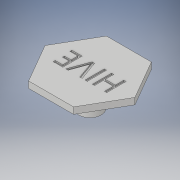
# Autodesk Inventor part: stand
Saved by Autodesk Inventor 2019 (Build 230136000, 136)
## iProperties
Created: 2018-06-01
Part Number: stand
Material: Generic
Document SubType Name: Modeling
Designer: HIVE
Density: 1 g/cm^3
Appearance: Default
Author: HIVE
## iProperties of the stored document stand_3DPrint.ipt
Created: 2018-06-01
Part Number: stand_3DPrint
Material: Generic
Document SubType Name: Modeling
Designer: HIVE
Density: 1 g/cm^3
Appearance: Default
Author: HIVE
Autodesk Inventor part; units mm, degrees
ref_plane "YZ Plane" through (0, 0, 0) normal (1, 0, 0) x (0, 1, 0)
ref_plane "XZ Plane" through (0, 0, 0) normal (0, 1, 0) x (-1, 0, 0)
ref_plane "XY Plane" through (0, 0, 0) normal (0, 0, 1) x (1, 0, 0)
sketch "Sketch1" plane through (0, 0, 0) normal (0, 1, 0) x (-1, 0, 0)
  circle A0 centre (0, 0) radius 35
  line L0 (17.5, -30.3109) -> (-17.5, -30.3109)
  line L1 (-17.5, -30.3109) -> (-35, 0)
  line L2 (-35, 0) -> (-17.5, 30.3109)
  line L3 (-17.5, 30.3109) -> (17.5, 30.3109)
  line L4 (17.5, 30.3109) -> (35, 0)
  line L5 (35, 0) -> (17.5, -30.3109)
  line L6 (16.3453, -28.3109) -> (-16.3453, -28.3109)
  line L7 (-16.3453, -28.3109) -> (-32.6906, 0)
  line L8 (-32.6906, 0) -> (-16.3453, 28.3109)
  line L9 (-16.3453, 28.3109) -> (16.3453, 28.3109)
  line L10 (16.3453, 28.3109) -> (32.6906, 0)
  line L11 (32.6906, 0) -> (16.3453, -28.3109)
  line L12 (0, 0) -> (-17.5, -30.3109)
  circle A1 centre (0, 0) radius 8.75
  line L13 (-22.7839, 7.707) -> (22.7839, 7.707) construction
  line L14 (22.7839, 7.707) -> (22.7839, -7.707) construction
  line L15 (22.7839, -7.707) -> (-22.7839, -7.707) construction
  line L16 (-22.7839, -7.707) -> (-22.7839, 7.707) construction
  line L17 (0, 0) -> (0, -28.3109) construction
  line L18 (1.5082, 8.619) -> (10.7506, 8.619) construction
  line L19 (-22.7839, 0) -> (22.7839, 0) construction
  line L20 (0, 7.707) -> (0, -7.707) construction
  line L21 (-20.822, 7.707) -> (-19.0548, 7.707)
  line L22 (-19.0548, 7.707) -> (-19.0548, 0.9167)
  line L23 (-19.0548, 0.9167) -> (-11.2904, 0.9167)
  line L24 (-11.2904, 0.9167) -> (-11.2904, 7.707)
  line L25 (-11.2904, 7.707) -> (-9.5372, 7.707)
  line L26 (-9.5372, 7.707) -> (-9.5372, -7.293)
  line L27 (-9.5372, -7.293) -> (-11.2904, -7.293)
  line L28 (-11.2904, -7.293) -> (-11.2904, -0.6557)
  line L29 (-11.2904, -0.6557) -> (-19.0548, -0.6557)
  line L30 (-19.0548, -0.6557) -> (-19.0548, -7.293)
  line L31 (-19.0548, -7.293) -> (-20.822, -7.293)
  line L32 (-20.822, -7.293) -> (-20.822, 7.707)
  line L33 (-5.6133, 7.707) -> (-3.8461, 7.707)
  line L34 (-3.8461, 7.707) -> (-3.8461, -7.293)
  line L35 (-3.8461, -7.293) -> (-5.6133, -7.293)
  line L36 (-5.6133, -7.293) -> (-5.6133, 7.707)
  line L37 (-1.7032, 7.707) -> (0.217, 7.707)
  line L38 (0.217, 7.707) -> (4.4053, -4.2456)
  spline S0 degree 2 poles (4.4053, -4.2456) (4.6279, -4.8301) (4.7253, -5.5815) knots 0 0 0 1 1 1
  line L39 (4.7253, -5.5815) -> (4.7671, -5.5815)
  spline S1 degree 2 poles (4.7671, -5.5815) (4.8506, -5.011) (5.1149, -4.2178) knots 0 0 0 1 1 1
  line L40 (5.1149, -4.2178) -> (9.3867, 7.707)
  line L41 (9.3867, 7.707) -> (11.2235, 7.707)
  line L42 (11.2235, 7.707) -> (5.6715, -7.3069)
  line L43 (5.6715, -7.3069) -> (3.7374, -7.3069)
  line L44 (3.7374, -7.3069) -> (-1.7032, 7.707)
  line L45 (13.3942, 7.707) -> (21.0194, 7.707)
  line L46 (21.0194, 7.707) -> (21.0194, 6.1208)
  line L47 (21.0194, 6.1208) -> (15.1613, 6.1208)
  line L48 (15.1613, 6.1208) -> (15.1613, 1.1254)
  line L49 (15.1613, 1.1254) -> (20.3654, 1.1254)
  line L50 (20.3654, 1.1254) -> (20.3654, -0.4469)
  line L51 (20.3654, -0.4469) -> (15.1613, -0.4469)
  line L52 (15.1613, -0.4469) -> (15.1613, -5.7067)
  line L53 (15.1613, -5.7067) -> (21.3534, -5.7067)
  line L54 (21.3534, -5.7067) -> (21.3534, -7.293)
  line L55 (21.3534, -7.293) -> (13.3942, -7.293)
  line L56 (13.3942, -7.293) -> (13.3942, 7.707)
  dimension "d0" = 70
  dimension "d2" = 17.5
  dimension "d1" = 2
  constraints: 34 end point, 7 midpoint, 5 coincident, 2 horizontal, 1 point on line, 34 other
  measures "d1" distance between parallel lines of L0 L6
extrude "Extrusion1" add sketch "Sketch1" against normal blind 3 contours L6 L7 L8 L9 L10 L11 | L35 L36 A1 | A1 L36 L33 | A1 L42 L43 | L40 L41 L42 A1 | L21 L22 L23 L24 L25 L26 L27 L28 L29 L30 L31 L32 | L45 L46 L47 L48 L49 L50 L51 L52 L53 L54 L55 L56
extrude "Extrusion3" add sketch "Sketch1" against normal blind 5 contours L5 L0 L1 L2 L3 L4
extrude "Extrusion4" add sketch "Sketch1" against normal blind 25 contours L34 L35 L12 | L12 L35 A1 L36 L33 L34 | L34 L33 A1 L40 S1 L39 S0 L38 L37 L44 L43 L12 L35 | L12 A1 L35 | L43 L44 L37 L38 S0 L39 S1 L40 A1 L42 | A1 L36 | L42 A1
extrude "Extrusion6" cut sketch "Sketch1" against normal blind 1 contours L34 L35 L12 | L12 L35 A1 L36 L33 L34 | L35 L36 A1 | A1 L36 L33 | L43 L44 L37 L38 S0 L39 S1 L40 A1 L42 | A1 L42 L43 | L40 L41 L42 A1 | L21 L22 L23 L24 L25 L26 L27 L28 L29 L30 L31 L32 | L45 L46 L47 L48 L49 L50 L51 L52 L53 L54 L55 L56
equation "\"d0\" = diam"
equation "\"d2\" = 0.25 * diam"
equation "\"d3\" = thickness"
equation "\"d9\" = 5 * d5"
equation "\"thickness\" = 3"
equation "\"diam\" = 70"
equation "\"d5\" = 5"
body "Solid1"
